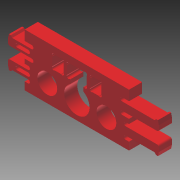
# Autodesk Inventor part: gantry5
Saved by Autodesk Inventor 2012 SP1 (Build 160190100, 190)
## iProperties
Created: 2011-10-14
Part Number: gantry5
Document SubType Name: Modeling
Designer: cramera
Density: 0.952 g/cm^3
Material: High Density Polyethylene
Mass: 40.2781 g
Surface Area: 182.857 cm^2
Volume: 42.309 cm^3
Autodesk Inventor part; units mm, degrees
ref_plane "YZ Plane" through (0, 0, 0) normal (1, 0, 0) x (0, 1, 0)
ref_plane "XZ Plane" through (0, 0, 0) normal (0, 1, 0) x (-1, 0, 0)
ref_plane "XY Plane" through (0, 0, 0) normal (0, 0, 1) x (1, 0, 0)
derived "skeleton.ipt"
sketch "STOCK_12MM" plane through (0, 0, 0) normal (0, 0, 1) x (1, 0, 0)
  line L0 (0, 0) -> (457.2, 0)
  line L1 (457.2, 0) -> (457.2, 914.4)
  line L2 (457.2, 914.4) -> (0, 914.4)
  line L3 (457.2, 914.4) -> (457.2, 0)
  line L4 (0, 914.4) -> (0, 0)
  constraints: 10 end point
sketch "THROUGH-CUT" plane through (0, 0, 0) normal (0, 0, 1) x (1, 0, 0)
  line L0 (95.8742, 445.4102) -> (95.8742, 453.2391)
  arc A0 (98.1193, 455.4842) -> (95.8742, 453.2391) centre (96.9967, 454.3617) ccw
  line L1 (98.1193, 455.4842) -> (103.7891, 455.4842)
  arc A1 (106.0342, 453.2391) -> (103.7891, 455.4842) centre (104.9117, 454.3617) ccw
  line L2 (106.0342, 453.2391) -> (106.0342, 445.4102)
  arc A2 (103.7891, 443.1652) -> (106.0342, 445.4102) centre (104.9117, 444.2877) ccw
  line L3 (103.7891, 443.1652) -> (98.1193, 443.1652)
  line L4 (89.7147, 443.1652) -> (89.7147, 439.5084)
  arc A3 (83.6822, 417.9531) -> (89.7147, 439.5084) centre (83.6822, 429.5749) ccw
  arc A4 (77.6497, 439.5084) -> (83.6822, 417.9531) centre (83.6822, 429.5749) ccw
  line L5 (77.6497, 439.5084) -> (77.6497, 443.1652)
  line L6 (77.6497, 443.1652) -> (77.0373, 443.1652)
  arc A5 (74.7922, 445.4102) -> (77.0373, 443.1652) centre (75.9147, 444.2877) ccw
  line L7 (74.7922, 445.4102) -> (74.7922, 453.2391)
  arc A6 (77.0373, 455.4842) -> (74.7922, 453.2391) centre (75.9147, 454.3617) ccw
  arc A7 (95.8742, 445.4102) -> (98.1193, 443.1652) centre (96.9967, 444.2877) ccw
  arc A8 (92.5722, 453.2391) -> (90.3271, 455.4842) centre (91.4497, 454.3617) ccw
  line L8 (92.5722, 453.2391) -> (92.5722, 445.4102)
  arc A9 (90.3271, 443.1652) -> (92.5722, 445.4102) centre (91.4497, 444.2877) ccw
  line L9 (90.3271, 443.1652) -> (89.7147, 443.1652)
  line L10 (63.5753, 455.4842) -> (69.2451, 455.4842)
  arc A10 (71.4902, 453.2391) -> (69.2451, 455.4842) centre (70.3677, 454.3617) ccw
  line L11 (71.4902, 453.2391) -> (71.4902, 445.4102)
  arc A11 (69.2451, 443.1652) -> (71.4902, 445.4102) centre (70.3677, 444.2877) ccw
  line L12 (69.2451, 443.1652) -> (63.5753, 443.1652)
  arc A12 (61.3302, 445.4102) -> (63.5753, 443.1652) centre (62.4527, 444.2877) ccw
  line L13 (61.3302, 445.4102) -> (61.3302, 453.2391)
  arc A13 (63.5753, 455.4842) -> (61.3302, 453.2391) centre (62.4527, 454.3617) ccw
  circle A14 centre (110.6696, 429.5754) radius 9.04
  circle A15 centre (56.6946, 429.5754) radius 9.04
  line L14 (77.0373, 455.4842) -> (90.3271, 455.4842)
  line L15 (36.0584, 420.7175) -> (39.2334, 420.7175)
  arc A16 (39.2334, 420.7175) -> (40.8209, 422.305) centre (39.2334, 422.305) ccw
  line L16 (40.8209, 422.305) -> (40.8209, 422.432)
  arc A17 (40.8209, 422.432) -> (39.2334, 424.0195) centre (39.2334, 422.432) ccw
  line L17 (39.2334, 424.0195) -> (36.0584, 424.0195)
  line L18 (36.0584, 424.0195) -> (27.2556, 424.0195)
  line L19 (27.2556, 424.0195) -> (24.6284, 424.0195)
  line L20 (24.6284, 424.0195) -> (23.3584, 422.4955)
  line L21 (23.3584, 422.4955) -> (21.6404, 422.4955)
  line L22 (21.6404, 422.4955) -> (20.8184, 426.095)
  line L23 (20.8184, 426.095) -> (20.8184, 429.8001)
  arc A18 (22.4059, 431.3855) -> (20.8184, 429.8001) centre (22.4059, 429.798) ccw
  line L24 (22.4059, 431.3855) -> (36.0584, 431.3855)
  line L25 (36.0584, 431.3855) -> (39.2334, 431.3855)
  arc A19 (39.2334, 431.3855) -> (40.8209, 432.973) centre (39.2334, 432.973) ccw
  line L26 (40.8209, 432.973) -> (40.8209, 433.1)
  arc A20 (40.8209, 433.1) -> (39.2334, 434.6875) centre (39.2334, 433.1) ccw
  line L27 (39.2334, 434.6875) -> (36.0584, 434.6875)
  line L28 (36.0584, 434.6875) -> (36.0584, 438.7515)
  line L29 (36.0584, 438.7515) -> (42.4084, 438.7515)
  arc A21 (42.4084, 438.7515) -> (43.9959, 440.339) centre (42.4084, 440.339) ccw
  line L30 (43.9959, 440.339) -> (43.9959, 440.466)
  arc A22 (43.9959, 440.466) -> (42.4084, 442.0535) centre (42.4084, 440.466) ccw
  line L31 (42.4084, 442.0535) -> (36.0584, 442.0535)
  line L32 (36.0584, 442.0535) -> (22.4059, 442.0535)
  arc A23 (20.8184, 443.6388) -> (22.4059, 442.0535) centre (22.4059, 443.641) ccw
  line L33 (20.8184, 443.6388) -> (20.8184, 447.3439)
  line L34 (20.8184, 447.3439) -> (21.6404, 450.9435)
  line L35 (21.6404, 450.9435) -> (23.3584, 450.9435)
  line L36 (23.3584, 450.9435) -> (24.6284, 449.4195)
  line L37 (24.6284, 449.4195) -> (27.2556, 449.4195)
  line L38 (27.2556, 449.4195) -> (36.0584, 449.4195)
  line L39 (36.0584, 449.4195) -> (42.4084, 449.4195)
  arc A24 (42.4084, 449.4195) -> (43.9959, 451.007) centre (42.4084, 451.007) ccw
  line L40 (43.9959, 451.007) -> (43.9959, 451.134)
  arc A25 (43.9959, 451.134) -> (42.4084, 452.7215) centre (42.4084, 451.134) ccw
  line L41 (42.4084, 452.7215) -> (36.0584, 452.7215)
  line L42 (36.0584, 452.7215) -> (36.0584, 461.835)
  line L43 (36.0584, 461.835) -> (131.3084, 461.835)
  line L44 (131.3084, 461.835) -> (131.3084, 452.7215)
  line L45 (131.3084, 452.7215) -> (124.9584, 452.7215)
  arc A26 (124.9584, 452.7215) -> (123.3709, 451.134) centre (124.9584, 451.134) ccw
  line L46 (123.3709, 451.134) -> (123.3709, 451.007)
  arc A27 (123.3709, 451.007) -> (124.9584, 449.4195) centre (124.9584, 451.007) ccw
  line L47 (124.9584, 449.4195) -> (131.3084, 449.4195)
  line L48 (131.3084, 449.4195) -> (154.7384, 449.4195)
  line L49 (154.7384, 449.4195) -> (156.0084, 450.9435)
  line L50 (156.0084, 450.9435) -> (157.7263, 450.9435)
  line L51 (157.7263, 450.9435) -> (158.5484, 447.3439)
  line L52 (158.5484, 447.3439) -> (158.5484, 443.6388)
  arc A28 (156.9609, 442.0535) -> (158.5484, 443.6388) centre (156.9609, 443.641) ccw
  line L53 (156.9609, 442.0535) -> (124.9584, 442.0535)
  arc A29 (124.9584, 442.0535) -> (123.3709, 440.466) centre (124.9584, 440.466) ccw
  line L54 (123.3709, 440.466) -> (123.3709, 440.339)
  arc A30 (123.3709, 440.339) -> (124.9584, 438.7515) centre (124.9584, 440.339) ccw
  line L55 (124.9584, 438.7515) -> (131.3084, 438.7515)
  line L56 (131.3084, 438.7515) -> (131.3084, 434.6875)
  line L57 (131.3084, 434.6875) -> (128.1334, 434.6875)
  arc A31 (128.1334, 434.6875) -> (126.5459, 433.1) centre (128.1334, 433.1) ccw
  line L58 (126.5459, 433.1) -> (126.5459, 432.973)
  arc A32 (126.5459, 432.973) -> (128.1334, 431.3855) centre (128.1334, 432.973) ccw
  line L59 (128.1334, 431.3855) -> (156.9609, 431.3855)
  arc A33 (158.5484, 429.8001) -> (156.9609, 431.3855) centre (156.9609, 429.798) ccw
  line L60 (158.5484, 429.8001) -> (158.5484, 426.095)
  line L61 (158.5484, 426.095) -> (157.7263, 422.4955)
  line L62 (157.7263, 422.4955) -> (156.0084, 422.4955)
  line L63 (156.0084, 422.4955) -> (154.7384, 424.0195)
  line L64 (154.7384, 424.0195) -> (131.3084, 424.0195)
  line L65 (131.3084, 424.0195) -> (128.1334, 424.0195)
  arc A34 (128.1334, 424.0195) -> (126.5459, 422.432) centre (128.1334, 422.432) ccw
  line L66 (126.5459, 422.432) -> (126.5459, 422.305)
  arc A35 (126.5459, 422.305) -> (128.1334, 420.7175) centre (128.1334, 422.305) ccw
  line L67 (128.1334, 420.7175) -> (131.3084, 420.7175)
  line L68 (131.3084, 420.7175) -> (131.3084, 413.7007)
  line L69 (131.3084, 413.7007) -> (36.0584, 413.7007)
  line L70 (36.0584, 413.7007) -> (36.0584, 420.7175)
  arc A36 (29.2913, 429.3527) -> (27.7038, 427.7652) centre (29.2913, 427.7652) ccw
  line L71 (27.7038, 427.7652) -> (27.7038, 427.6382)
  arc A37 (27.7038, 427.6382) -> (29.2913, 426.0507) centre (29.2913, 427.6382) ccw
  line L72 (29.2913, 426.0507) -> (39.2322, 426.0507)
  arc A38 (39.2322, 426.0507) -> (40.8197, 427.6382) centre (39.2322, 427.6382) ccw
  line L73 (40.8197, 427.6382) -> (40.8197, 427.7652)
  arc A39 (40.8197, 427.7652) -> (39.2322, 429.3527) centre (39.2322, 427.7652) ccw
  line L74 (39.2322, 429.3527) -> (29.2913, 429.3527)
  arc A40 (39.2322, 444.0847) -> (40.8197, 445.6695) centre (39.2322, 445.6722) ccw
  line L75 (40.8197, 445.6695) -> (40.8197, 445.7992)
  arc A41 (40.8197, 445.7992) -> (39.2322, 447.3867) centre (39.2322, 445.7992) ccw
  line L76 (39.2322, 447.3867) -> (29.2913, 447.3867)
  arc A42 (29.2913, 447.3867) -> (27.7038, 445.7992) centre (29.2913, 445.7992) ccw
  line L77 (27.7038, 445.7992) -> (27.7038, 445.6722)
  arc A43 (27.7038, 445.6722) -> (29.2913, 444.0847) centre (29.2913, 445.6722) ccw
  line L78 (29.2913, 444.0847) -> (39.2322, 444.0847)
  dimension "d3" = 18.08
  dimension "d4" = 18.08
  constraints: 158 end point, 84 point on circle, 44 centre point
  measures "d3" diameter of A15
  measures "d4" diameter of A14
extrude "Extrusion1" add sketch "THROUGH-CUT" along normal blind 12
equation "\"d4\" = d3"
equation "\"d1\" = StockThickness"
equation "\"StockThickness\" = 12"
body "Solid1"
